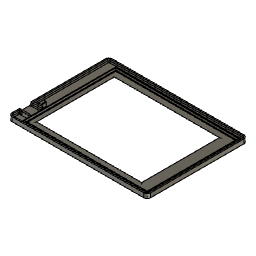
Soldered Inkplate 6plus v1.2.0. Top v1.2.1. (Autodesk Fusion 360 design; units mm, degrees)
Autodesk Fusion 360 part; units mm, degrees
sketch "Sketch1" plane through (0, 0, 0) normal (0, 0, 1) x (1, 0, 0)
  line L0 (80.7, 58.4) -> (-80.7, 58.4)
  line L1 (-80.7, 58.4) -> (-80.7, -58.4)
  line L2 (-80.7, -58.4) -> (80.7, -58.4)
  line L3 (80.7, -58.4) -> (80.7, 58.4)
  line L4 (80.7, 58.4) -> (-80.7, -58.4) construction
  line L5 (-80.7, 58.4) -> (80.7, -58.4) construction
  line L6 (61.2, 45.3) -> (-61.2, 45.3)
  line L7 (-61.2, 45.3) -> (-61.2, -45.3)
  line L8 (-61.2, -45.3) -> (61.2, -45.3)
  line L9 (61.2, -45.3) -> (61.2, 45.3)
  line L10 (61.2, 45.3) -> (-61.2, -45.3) construction
  line L11 (-61.2, 45.3) -> (61.2, -45.3) construction
  dimension "d1" = 116.8
  dimension "d2" = 161.4
  dimension "d3" = 122.4
  dimension "d4" = 90.6
  constraint horizontal L0
  constraint perpendicular L0 L1
  constraint parallel L0 L2
  constraint parallel L1 L3
  constraint coincident L4 origin
  constraint coincident L5 origin
  constraint horizontal L6
  constraint perpendicular L6 L7
  constraint parallel L6 L8
  constraint parallel L7 L9
  constraint coincident L10 origin
  constraint coincident L11 origin
  measures "d1" distance of L0.end L1.end
  measures "d2" distance of L1.end L2.end
  measures "d3" distance of L7.end L8.end
  measures "d4" distance of L6.end L7.end
extrude "Extrude1" add sketch "Sketch1" along normal blind 5
sketch "Sketch2" plane through (0, 0, 5) normal (0, 0, 1) x (-1, 0, 0)
  line L0 (-61.2, -45.3) -> (-61.2, 45.3)
  line L1 (-61.2, 45.3) -> (61.2, 45.3)
  line L2 (61.2, 45.3) -> (61.2, -45.3)
  line L3 (61.2, -45.3) -> (-61.2, -45.3)
  line L4 (-80.7, 58.4) -> (-80.7, -58.4)
  line L5 (-80.7, -58.4) -> (80.7, -58.4)
  line L6 (80.7, -58.4) -> (80.7, 58.4)
  line L7 (80.7, 58.4) -> (-80.7, 58.4)
  line L8 (79.2, 56.9) -> (-79.2, 56.9)
  line L9 (-79.2, 56.9) -> (-79.2, -56.9)
  line L10 (-79.2, -56.9) -> (79.2, -56.9)
  line L11 (79.2, -56.9) -> (79.2, 56.9)
  line L12 (79.2, 56.9) -> (-79.2, -56.9) construction
  line L13 (-79.2, 56.9) -> (79.2, -56.9) construction
  dimension "d7" = 1.5
  dimension "d8" = 1.5
  constraint horizontal L8
  constraint perpendicular L8 L9
  constraint parallel L8 L10
  constraint parallel L9 L11
  constraint coincident L12 origin
  constraint coincident L13 origin
  measures "d7" distance of L7 L8
  measures "d8" distance of L6 L11
extrude "Extrude2" cut sketch "Sketch2" against normal blind 4 contours L8 L9 L10 L11
chamfer "Chamfer1" distance 1 distance2 2 4 edges at (0, -45.3, 0) (-61.2, 0, 0) (61.2, 0, 0) (0, 45.3, 0) measured on face at (-20.4, -45.3, 0.6667) measured on face at (-61.2, 15.1, 0.3333) measured on face at (61.2, -15.1, 0.3333) measured on face at (20.4, 45.3, 0.6667)
fillet "Fillet1" radius 4 4 edges at (-80.7, 58.4, 2.5) (80.7, 58.4, 2.5) (80.7, -58.4, 2.5) (-80.7, -58.4, 2.5)
sketch "Sketch3" plane through (0, 0, 1) normal (0, 0, 1) x (-1, 0, 0)
  line L0 (61.2, 45.3) -> (61.2, -45.3)
  line L1 (61.2, -45.3) -> (-61.2, -45.3)
  line L2 (-61.2, -45.3) -> (-61.2, 45.3)
  line L3 (-61.2, 45.3) -> (61.2, 45.3)
  line L4 (79.2, -56.9) -> (79.2, 56.9)
  line L5 (79.2, 56.9) -> (-79.2, 56.9)
  line L6 (-79.2, 56.9) -> (-79.2, -56.9)
  line L7 (-79.2, -56.9) -> (79.2, -56.9)
  line L8 (68.2, 49) -> (68.2, 10) construction
  line L9 (61.2, 45.4) -> (91.0254, 45.4) construction
  line L10 (76.7, 58.4) -> (-76.7, 58.4)
  line L11 (65.2059, 47.4) -> (83.4218, 47.4) construction
  line L12 (66.5823, 32.4) -> (83.713, 32.4) construction
  line L13 (65.5907, 30.4) -> (91.8883, 30.4) construction
  line L14 (76, 48.6711) -> (76, 29) construction
  line L15 (68.2, 47.4) -> (76, 47.4)
  line L16 (76, 47.4) -> (76, 30.4)
  line L17 (76, 30.4) -> (68.2, 30.4)
  line L18 (68.2, 30.4) -> (68.2, 47.4)
  line L19 (76, 30.4) -> (79.2, 30.4)
  line L20 (79.2, 30.4) -> (79.2, 32.4)
  line L21 (79.2, 32.4) -> (76, 32.4)
  line L22 (76, 32.4) -> (76, 30.4)
  dimension "d15" = 11
  dimension "d16" = 13
  dimension "d17" = 2
  dimension "d18" = 13
  dimension "d19" = 2
  dimension "d20" = 3.2
  constraint vertical L8
  constraint coincident L0 L9.start
  constraint perpendicular L8 L9
  constraint perpendicular L4 L11
  constraint horizontal L12
  constraint perpendicular L8 L13
  constraint perpendicular L13 L14
  constraint horizontal L15
  constraint vertical L16
  constraint horizontal L17
  constraint vertical L18
  constraint coincident L13 L16.end
  constraint coincident L14 L16.end
  constraint coincident L11 L15.start
  constraint coincident L8 L15.start
  constraint horizontal L19
  constraint vertical L20
  constraint horizontal L21
  constraint vertical L22
  constraint coincident L12 L20.end
  constraint coincident L4 L20.end
  measures "d15" distance of L4 L8
  measures "d16" distance of L9 L10
  measures "d17" distance of L9 L11
  measures "d18" distance of L9 L12
  measures "d19" distance of L12 L13
  measures "d20" distance of L4 L14
extrude "Extrude3" add sketch "Sketch3" along normal blind 4 contours L4 L16 L19 L20 L21 L22 | L15 L16 L17 L18 L22
sketch "Sketch4" plane through (-80.7, 0, 0) normal (-1, 0, 0) x (0, -1, 0)
  line L0 (54.4, 0) -> (54.4, 5)
  line L1 (54.4, 5) -> (-54.4, 5)
  line L2 (-54.4, 5) -> (-54.4, 0)
  line L3 (-54.4, 0) -> (54.4, 0)
  line L4 (45.4, 8) -> (45.4, -6) construction
  line L5 (58.4, 0) -> (58.4, 5)
  line L6 (45.4, 5) -> (32.4, 5)
  line L7 (32.4, 5) -> (32.4, 2)
  line L8 (32.4, 2) -> (45.4, 2)
  line L9 (45.4, 2) -> (45.4, 5)
  dimension "d23" = 13
  dimension "d24" = 13
  dimension "d25" = 3
  constraint perpendicular L3 L4
  constraint horizontal L6
  constraint vertical L7
  constraint horizontal L8
  constraint vertical L9
  constraint coincident L4 L6.start
  constraint coincident L1 L6.start
  measures "d23" distance of L4 L5
  measures "d24" distance of L6.start L6.end
  measures "d25" distance of L6.start L8.end
extrude "Extrude4" cut sketch "Sketch4" against normal blind 12.5 contours L1 L6 L7 L8 L9
sketch "Sketch5" plane through (0, 0, 1) normal (0, 0, 1) x (-1, 0, 0)
  line L0 (79.2, 30.4) -> (68.2, 30.4)
  line L1 (68.2, 30.4) -> (68.2, 47.4)
  line L2 (68.2, 47.4) -> (76, 47.4)
  line L3 (76, 47.4) -> (76, 32.4)
  line L4 (76, 32.4) -> (79.2, 32.4)
  line L5 (79.2, 32.4) -> (79.2, 56.9)
  line L6 (79.2, 56.9) -> (-79.2, 56.9)
  line L7 (-79.2, 56.9) -> (-79.2, -56.9)
  line L8 (-79.2, -56.9) -> (79.2, -56.9)
  line L9 (79.2, -56.9) -> (79.2, 30.4)
  line L10 (61.2, 45.3) -> (61.2, -45.3)
  line L11 (61.2, -45.3) -> (-61.2, -45.3)
  line L12 (-61.2, -45.3) -> (-61.2, 45.3)
  line L13 (-61.2, 45.3) -> (61.2, 45.3)
  line L14 (68.2, 53.9) -> (-76.2, 53.9)
  line L15 (-76.2, 53.9) -> (-76.2, -53.9)
  line L16 (-76.2, -53.9) -> (68.2, -53.9)
  line L17 (68.2, -53.9) -> (68.2, 53.9)
  line L18 (68.2, 53.9) -> (-76.2, -53.9) construction
  line L19 (-76.2, 53.9) -> (68.2, -53.9) construction
  line L20 (66.2, 51.9) -> (-74.2, 51.9)
  line L21 (-74.2, 51.9) -> (-74.2, -51.9)
  line L22 (-74.2, -51.9) -> (66.2, -51.9)
  line L23 (66.2, -51.9) -> (66.2, 51.9)
  line L24 (66.2, 51.9) -> (-74.2, -51.9) construction
  line L25 (-74.2, 51.9) -> (66.2, -51.9) construction
  point P0 (-4, 0)
  dimension "d28" = 144.4
  dimension "d29" = 107.8
  dimension "d30" = 15
  dimension "d31" = 2
  dimension "d32" = 2
  dimension "d33" = 8.6
  constraint horizontal L14
  constraint perpendicular L14 L15
  constraint parallel L14 L16
  constraint parallel L15 L17
  constraint horizontal L20
  constraint perpendicular L20 L21
  constraint parallel L20 L22
  constraint parallel L21 L23
  constraint coincident L24 P0
  constraint coincident L25 P0
  constraint midpoint L18 P0
  measures "d28" distance of L15.end L16.end
  measures "d29" distance of L14.end L15.end
  measures "d30" distance of L12 L15
  measures "d31" distance of L14 L20
  measures "d32" distance of L17 L23
  measures "d33" distance of L13 L14
extrude "Extrude5" add sketch "Sketch5" along normal blind 2.3 contours L1 L14 L15 L16 L17
fillet "Fillet3" radius 2 2 edges at (-79.95, -32.4, 2) (-79.95, -45.4, 2)
sketch "Sketch6" plane through (0, 0, 1) normal (0, 0, 1) x (-1, 0, 0)
  line L0 (68.2, 53.9) -> (68.2, 47.4)
  line L1 (68.2, 47.4) -> (76, 47.4)
  line L2 (76, 47.4) -> (76, 32.4)
  line L3 (76, 32.4) -> (79.2, 32.4)
  line L4 (79.2, 32.4) -> (79.2, 56.9)
  line L5 (79.2, 56.9) -> (-79.2, 56.9)
  line L6 (-79.2, 56.9) -> (-79.2, -56.9)
  line L7 (-79.2, -56.9) -> (79.2, -56.9)
  line L8 (79.2, -56.9) -> (79.2, 30.4)
  line L9 (79.2, 30.4) -> (68.2, 30.4)
  line L10 (68.2, 30.4) -> (68.2, -53.9)
  line L11 (68.2, -53.9) -> (-76.2, -53.9)
  line L12 (-76.2, -53.9) -> (-76.2, 53.9)
  line L13 (-76.2, 53.9) -> (68.2, 53.9)
  line L14 (76, 47.4) -> (79.2, 47.4)
  line L15 (79.2, 47.4) -> (79.2, 32.4)
  line L16 (79.2, 32.4) -> (76, 32.4)
  line L17 (76, 32.4) -> (76, 47.4)
  constraint horizontal L14
  constraint vertical L15
  constraint horizontal L16
  constraint vertical L17
  constraint coincident L3.end L4.start
  constraint coincident L1.end L2.start
extrude "Extrude6" add sketch "Sketch6" along normal blind 1 contours L2 L3 L4 L14 L15 L16 L17
fillet "Fillet2" radius 1 3 edges at (-72.1, -45.4, 2) (-73.7, -32.4, 2) (-68.2, -38.9, 2)
ref_plane "WorkPlane1" through (0, 0, 2.5) normal (0, 0, 1) x (1, 0, 0)
sketch "Sketch7" plane through (0, 0, 2.5) normal (0, 0, 1) x (1, 0, 0)
  line L0 (-79.2, -30.4) -> (-78.2, -30.4)
  line L1 (-78.2, -30.4) -> (-78.2, 54.9)
  line L2 (-78.2, 56.9) -> (-79.2, 56.9)
  line L3 (-79.2, 56.9) -> (-79.2, -30.4)
  line L4 (-79.2, 56.9) -> (79.2, 56.9)
  line L5 (-79.2, 56.9) -> (79.2, 56.9)
  line L6 (79.2, 56.9) -> (79.2, 55.9)
  line L7 (77.2, 55.9) -> (-77.2, 55.9)
  line L8 (-79.2, 55.9) -> (-79.2, 56.9)
  line L9 (79.2, 56.9) -> (79.2, -56.9)
  line L10 (79.2, 56.9) -> (78.2, 56.9)
  line L11 (78.2, 54.9) -> (78.2, -54.9)
  line L12 (78.2, -56.9) -> (79.2, -56.9)
  line L13 (79.2, -56.9) -> (79.2, 56.9)
  line L14 (79.2, -56.9) -> (-79.2, -56.9)
  line L15 (79.2, -56.9) -> (-79.2, -56.9)
  line L16 (-79.2, -56.9) -> (-79.2, -55.9)
  line L17 (-77.2, -55.9) -> (77.2, -55.9)
  line L18 (79.2, -55.9) -> (79.2, -56.9)
  line L19 (-79.2, -56.9) -> (-78.2, -56.9)
  line L20 (-78.2, -54.9) -> (-78.2, -47.4)
  line L21 (-78.2, -47.4) -> (-79.2, -47.4)
  line L22 (-79.2, -47.4) -> (-79.2, -56.9)
  line L23 (-79.2, -47.4) -> (-76, -47.4)
  line L24 (-68.2, -30.4) -> (-79.2, -30.4)
  arc A0 (-78.2, -54.9) -> (-77.2, -55.9) centre (-77.2, -54.9) ccw
  arc A1 (77.2, -55.9) -> (78.2, -54.9) centre (77.2, -54.9) ccw
  arc A2 (78.2, 54.9) -> (77.2, 55.9) centre (77.2, 54.9) ccw
  arc A3 (-77.2, 55.9) -> (-78.2, 54.9) centre (-77.2, 54.9) ccw
  dimension "d41" = 1
  dimension "d42" = 1
  dimension "d43" = 1
  dimension "d44" = 1
  dimension "d45" = 1
  dimension "d48" = 1
  dimension "d49" = 1
  dimension "d50" = 1
  dimension "d51" = 1
  constraint horizontal L0
  constraint vertical L1
  constraint horizontal L2
  constraint vertical L3
  constraint coincident L2.start L4
  constraint coincident L2.end L3.start
  constraint horizontal L5
  constraint vertical L6
  constraint horizontal L7
  constraint vertical L8
  constraint coincident L6.end L9
  constraint horizontal L10
  constraint vertical L11
  constraint horizontal L12
  constraint vertical L13
  constraint coincident L4.end L5.end
  constraint coincident L12.start L14
  constraint horizontal L15
  constraint vertical L16
  constraint horizontal L17
  constraint vertical L18
  constraint coincident L9.end L12.end
  constraint coincident L14.end L15.end
  constraint horizontal L19
  constraint vertical L20
  constraint horizontal L21
  constraint vertical L22
  constraint coincident L0.start L3.end
  constraint coincident L21.end L22.start
  constraint coincident L19.end L20
  constraint coincident L16.end L17
  constraint tangent L20 A0
  constraint tangent L17 A0
  constraint coincident L12.start L11
  constraint coincident L18.start L17
  constraint tangent L11 A1
  constraint tangent L17 A1
  constraint coincident L6.end L7
  constraint coincident L10.end L11
  constraint tangent L7 A2
  constraint tangent L11 A2
  constraint coincident L8.start L7
  constraint coincident L2.start L1
  constraint tangent L7 A3
  constraint tangent L1 A3
  measures "d41" distance of L0.end L0.start
  measures "d42" distance of L2.end L8.start
  measures "d43" distance of L4.end L10.end
  measures "d44" distance of L15 L17
  measures "d45" distance of L14.end L19.end
  measures "d48" radius of A0
  measures "d49" radius of A1
  measures "d50" radius of A2
  measures "d51" radius of A3
extrude "Extrude7" add sketch "Sketch7" along normal blind 2.5
chamfer "Chamfer2" distance 1.5 distance2 1.5 9 edges at (-78.2, 12.25, 2.5) (-77.9071, 55.6071, 2.5) (0, 55.9, 2.5) (77.9071, 55.6071, 2.5) (78.2, 0, 2.5) (77.9071, -55.6071, 2.5) (0, -55.9, 2.5) (-77.9071, -55.6071, 2.5) (-78.2, -51.15, 2.5) measured on face at (-78.2, -1.9667, 3.3333) measured on face at (-25.7333, -56.5667, 2.5) measured on face at (-25.7333, -56.5667, 2.5) measured on face at (-25.7333, -56.5667, 2.5) measured on face at (78.2, 18.3, 3.3333) measured on face at (-25.7333, -56.5667, 2.5) measured on face at (-25.7333, -56.5667, 2.5) measured on face at (-25.7333, -56.5667, 2.5) measured on face at (-78.2, -52.4, 3.3333)
chamfer "Chamfer3" distance 1.2 distance2 1.2 4 edges at (-66.2, 0, 3.3) (4, 51.9, 3.3) (4, -51.9, 3.3) (74.2, 0, 3.3) measured on face at (-66.8667, -10.1333, 3.3) measured on face at (-66.8667, -10.1333, 3.3) measured on face at (-66.8667, -10.1333, 3.3) measured on face at (-66.8667, -10.1333, 3.3)
chamfer "Chamfer4" distance 1 distance2 1 9 edges at (-78.2, 12.25, 5) (-77.9071, 55.6071, 5) (0, 55.9, 5) (77.9071, 55.6071, 5) (78.2, 0, 5) (77.9071, -55.6071, 5) (0, -55.9, 5) (-77.9071, -55.6071, 5) (-78.2, -51.15, 5) measured on face at (-25.5667, -56.7333, 5) measured on face at (-25.5667, -56.7333, 5) measured on face at (-25.5667, -56.7333, 5) measured on face at (-25.5667, -56.7333, 5) measured on face at (-25.5667, -56.7333, 5) measured on face at (-25.5667, -56.7333, 5) measured on face at (-25.5667, -56.7333, 5) measured on face at (-25.5667, -56.7333, 5) measured on face at (-25.5667, -56.7333, 5)
sketch "Sketch9" plane through (0, 0, 1) normal (0, 0, 1) x (-1, 0, 0)
  line L0 (68.2, 47.4) -> (79.2, 47.4)
  line L1 (79.2, 47.4) -> (79.2, 56.9)
  line L2 (79.2, 56.9) -> (-79.2, 56.9)
  line L3 (-79.2, 56.9) -> (-79.2, -56.9)
  line L4 (-79.2, -56.9) -> (79.2, -56.9)
  line L5 (79.2, -56.9) -> (79.2, 30.4)
  line L6 (79.2, 30.4) -> (68.2, 30.4)
  line L7 (68.2, 30.4) -> (68.2, -53.9)
  line L8 (68.2, -53.9) -> (-76.2, -53.9)
  line L9 (-76.2, -53.9) -> (-76.2, 53.9)
  line L10 (-76.2, 53.9) -> (68.2, 53.9)
  line L11 (68.2, 53.9) -> (68.2, 47.4)
  line L12 (83, 29.4) -> (82, 29.4) construction
  line L13 (82, 29.4) -> (64, 29.4) construction
  line L14 (74.7, 29.4) -> (71.2, 29.4)
  line L15 (71.2, 29.4) -> (71.2, 23.9)
  line L16 (71.2, 23.9) -> (74.7, 23.9)
  line L17 (74.7, 23.9) -> (74.7, 29.4)
  line L18 (80.7, -54.4) -> (80.7, 32.4)
  dimension "d67" = 1
  dimension "d68" = 3.5
  dimension "d69" = 5.5
  dimension "d70" = 6
  constraint horizontal L12
  constraint parallel L12 L13
  constraint horizontal L14
  constraint vertical L15
  constraint horizontal L16
  constraint vertical L17
  constraint coincident L13 L14.start
  measures "d67" distance of L6 L13
  measures "d68" distance of L14.start L14.end
  measures "d69" distance of L14.start L16.end
  measures "d70" distance of L17 L18
extrude "Extrude9" add sketch "Sketch9" along normal blind 4.6 contours L14 L15 L16 L17
chamfer "Chamfer5" distance 0.5 angle 45 1 edges at (-71.2, -26.65, 5.6)
